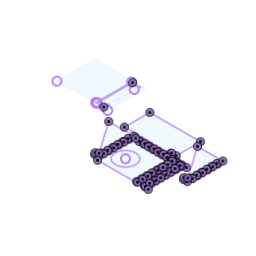
Verkefni2 (Autodesk Fusion 360 design; units mm, degrees)
Autodesk Fusion 360 part; units mm, degrees
note: some values were not read from the file. Chosen so that the rebuilt part matches the saved one: that a step has no effect.
sketch "haldari sketch" plane through (0, 0, 0) normal (1, 0, 0) x (0, 1, 0) in component "Fótur"
  line L0 (0, 0) -> (140, 0)
  line L1 (140, 0) -> (140, 100)
  line L2 (140, 100) -> (12.8948, 11)
  line L3 (12.8948, 11) -> (6.3582, 20.3352)
  line L4 (6.3582, 20.3352) -> (0, 15)
  line L5 (0, 15) -> (0, 0)
  dimension "d8" = 140
  dimension "d9" = 100
  dimension "d10" = 55
  dimension "d13" = 50
  dimension "d141" = 11
  dimension "d142" = 15
  constraint coincident L0.start L5.end
  constraint horizontal L0
  constraint perpendicular L0 L1
  constraint perpendicular L2 L3
  constraint perpendicular L0 L5
  measures "d8" distance of L0.start L0.end
  measures "d9" distance of L0.end L1.end
  measures "d10" angle of L1 L2
  measures "d13" angle of L4 L5
  measures "d141" distance of L0 L2.end
  measures "d142" distance of L0.start L4.end
extrude "Extrude6" add sketch "haldari sketch" along normal blind 4 makes body 1 in component "Fótur"
sketch "fingerhaldari sketch" plane through (4, 0, 0) normal (1, 0, 0) x (0, 1, 0) in component "Fótur"
  line L0 (0, 15) -> (0, 0)
  line L1 (0, 0) -> (140, 0)
  line L2 (140, 0) -> (140, 100)
  line L3 (140, 100) -> (12.8948, 11)
  line L4 (12.8948, 11) -> (6.3582, 20.3352)
  line L5 (6.3582, 20.3352) -> (0, 15)
  line L6 (90, 0) -> (90, 4)
  line L7 (90, 4) -> (0, 4)
  line L8 (0, 4) -> (0, 0)
  line L9 (20, 0) -> (40, 0)
  line L10 (40, 0) -> (40, 4)
  line L11 (40, 4) -> (20, 4)
  line L12 (20, 4) -> (20, 0)
  dimension "d72" = 4
  dimension "d73" = 20
  dimension "d79" = 20
  constraint vertical L6
  constraint horizontal L7
  constraint vertical L8
  constraint coincident L0.end L1.start
  constraint horizontal L9
  constraint vertical L10
  constraint horizontal L11
  constraint vertical L12
  constraint coincident L7 L10.end
  constraint coincident L1 L9.start
  measures "d72" distance of L0.end L7.end
  measures "d73" distance of L8 L12
  measures "d79" distance of L10.end L11.end
extrude "Extrude8" cut sketch "fingerhaldari sketch" against normal blind 4 contours L1 L7 L9 L10 L11 L12 bodies 1 in component "Fótur"
pattern_linear "R-Pattern2" count 3 spacing 40 along (0, 1, 0) of "Extrude8" in component "Fótur"
sketch "Sketch1" plane through (-1, 0, 0.1216) normal (0, 0, -1) x (1, 0, 0) in component "Botn"
  line L0 (32, -20) -> (36, -20)
  line L1 (36, -20) -> (36, 0)
  line L2 (36, 0) -> (32, 0)
  line L3 (32, 0) -> (32, -20)
  line L4 (-149, 4) -> (51, 4)
  line L5 (51, 4) -> (51, -146)
  line L6 (51, -146) -> (-149, -146)
  line L7 (-149, -146) -> (-149, 4)
  line L8 (1, 0) -> (1, -140)
  line L9 (1, 0) -> (5, 0)
  dimension "d96" = 200
  dimension "d97" = 150
  dimension "d98" = 150
  dimension "d99" = 4
  constraint horizontal L4
  constraint vertical L5
  constraint horizontal L6
  constraint vertical L7
  measures "d96" distance of L4.start L4.end
  measures "d97" distance of L4.start L6.end
  measures "d98" distance of L7 L8
  measures "d99" distance of L4 L9
extrude "Extrude1" add sketch "Sketch1" against normal blind 4 separate body makes body 2 in component "Botn"
combine "Combine1" operation cut target body 2 tool bodies 1 body 1 seen with x (1, 0, 0) y (0, 1, 0) z (0, 0, 1) at (31, 0, 0.1216) keep tools in component "Botn"
combine "Combine2" operation cut target body 2 tool bodies 1 keep tools in component "Botn"
combine "Combine3" operation cut target body 2 tool bodies 1 keep tools in component "Botn"
sketch "Sketch2" plane through (0, 0, 4.1216) normal (0, 0, 1) x (-1, 0, 0)
  line L0 (-31, -120) -> (-31, -140)
  line L1 (-35, -140) -> (-35, -120)
  line L2 (-35, -120) -> (-31, -120)
  line L3 (-31, -100) -> (-35, -100)
  line L4 (-35, -100) -> (-35, -80)
  line L5 (-35, -80) -> (-31, -80)
  line L6 (-31, -80) -> (-31, -100)
  line L7 (-31, -60) -> (-35, -60)
  line L8 (-35, -60) -> (-35, -40)
  line L9 (-35, -40) -> (-31, -40)
  line L10 (-31, -40) -> (-31, -60)
  line L11 (150, -146) -> (150, 4)
  line L12 (150, 4) -> (-50, 4)
  line L13 (-50, 4) -> (-50, -146)
  line L14 (-50, -146) -> (150, -146)
  line L15 (-31, -20) -> (-35, -20)
  line L16 (-35, -20) -> (-35, 0)
  line L17 (-4, -140) -> (-4, 0)
  line L18 (-4, 0) -> (0, 0)
  line L19 (0, 0) -> (0, -140)
  line L20 (0, -140) -> (-4, -140)
  line L21 (-31, -140) -> (-35, -140)
  line L22 (-35, 0) -> (-31, 0)
  line L23 (-31, 0) -> (-31, -20)
sketch "Sketch3" plane through (0, 146, 0) normal (0, 1, 0) x (-1, 0, 0)
  line L0 (-50, 0.1216) -> (150, 0.1216)
  line L1 (150, 0.1216) -> (150, 4.1216)
  line L2 (150, 4.1216) -> (-50, 4.1216)
  line L3 (-50, 4.1216) -> (-50, 0.1216)
  line L4 (-31.8182, 0.1216) -> (-13.6364, 0.1216)
  line L5 (-13.6364, 0.1216) -> (-13.6364, 4.1216)
  line L6 (-13.6364, 4.1216) -> (-31.8182, 4.1216)
  line L7 (-31.8182, 4.1216) -> (-31.8182, 0.1216)
  dimension "d133" = 18.1818
  dimension "d134" = 18.1818
  constraint horizontal L4
  constraint vertical L5
  constraint horizontal L6
  constraint vertical L7
  constraint coincident L2 L5.end
  constraint coincident L0 L4.start
  measures "d133" distance of L3 L7
  measures "d134" distance of L4.start L4.end
extrude "Extrude4" cut sketch "Sketch3" against normal blind 4 contours L0 L2 L4 L5 L6 L7 bodies 2 in component "Botn"
pattern_linear "R-Pattern2'" count 5 spacing 36.3636 along (-1, 0, 0) of "Extrude4" in component "Botn"
sketch "Sketch4" plane through (0, 0, 0.1216) normal (0, 0, -1) x (1, 0, 0)
  circle A0 centre (-100, -56) radius 40
  line L0 (-150, -146) -> (-150, 4)
  line L1 (-150, 4) -> (50, 4)
  dimension "d143" = 80
  dimension "d144" = 50
  dimension "d145" = 60
  measures "d143" diameter of A0
  measures "d144" distance of A0.centre L0
  measures "d145" distance of A0.centre L1
extrude "Extrude5" cut sketch "Sketch4" against normal blind 4 bodies 2 in component "Botn"
sketch "Sketch1 (2)" plane through (0, 146, 0) normal (0, 1, 0) x (-1, 0, 0) in component "Hlið"
  line L0 (-31.8182, 0.1216) -> (-31.8182, 4.1216)
  line L1 (-31.8182, 4.1216) -> (-50, 4.1216)
  line L2 (-50, 4.1216) -> (-50, 0.1216)
  line L3 (-50, 0.1216) -> (-31.8182, 0.1216)
  line L4 (-50, 0.1216) -> (150, 0.1216)
  line L5 (150, 0.1216) -> (150, 100.1216)
  line L6 (150, 100.1216) -> (-50, 100.1216)
  line L7 (-50, 100.1216) -> (-50, 0.1216)
  dimension "d148" = 200
  dimension "d149" = 100
  constraint horizontal L4
  constraint vertical L5
  constraint horizontal L6
  constraint vertical L7
  constraint coincident L2.end L3.start
  measures "d148" distance of L2.end L4.end
  measures "d149" distance of L2.end L6.end
extrude "Extrude1'" add sketch "Sketch1 (2)" against normal blind 4 separate body contours L0 L1 L4 L5 L6 L7 makes body 3 in component "Hlið"
combine "Combine1'" [no effect] in component "Hlið"
move_body "Move1" bodies 2 to x (1, 0, 0) y (0, 1, 0) z (0, 0, 1) at (70, -190, 0) in component "Botn"
move_body "Align1" bodies 1 to x (0, 0, 1) y (0, 1, 0) z (-1, 0, 0) at (50, 0, 4.1216) in component "Fótur"
move_body "Align2" bodies 1 to x (1, 0, 0) y (0, 1, 0) z (0, 0, 1) at (0, 0, -4.1216) in component "Fótur"
move_body "Align1'" bodies 3 to x (1, 0, 0) y (0, 0, -1) z (0, 1, 0) at (0, 91.8784, 146.1216) in component "Hlið"
move_body "Move1'" bodies 3 to x (1, 0, 0) y (0, 1, 0) z (0, 0, 1) at (0, -120, 0) in component "Hlið"
move_body "Move2" bodies 3 to x (1, 0, 0) y (0, 1, 0) z (0, 0, 1) at (10, 0, 0) in component "Hlið"
sketch "Sketch1 (3)" plane through (0, 0, 4.1216) normal (0, 0, 1) x (-1, 0, 0) in component "Cam Layer"
  circle A0 centre (-250, 134) radius 40
  line L0 (-381, 170) -> (-385, 170)
  line L1 (-385, 170) -> (-385, 190)
  line L2 (-385, 190) -> (-381, 190)
  line L3 (-381, 190) -> (-381, 170)
  line L4 (-236.3636, 44) -> (-236.3636, 48)
  line L5 (-236.3636, 48) -> (-218.1818, 48)
  line L6 (-218.1818, 48) -> (-218.1818, 44)
  line L7 (-218.1818, 44) -> (-200, 44)
  line L8 (-200, 44) -> (-200, 194)
  line L9 (-200, 194) -> (-400, 194)
  line L10 (-400, 194) -> (-400, 44)
  line L11 (-400, 44) -> (-381.8182, 44)
  line L12 (-381.8182, 44) -> (-381.8182, 48)
  line L13 (-381.8182, 48) -> (-363.6364, 48)
  line L14 (-363.6364, 48) -> (-363.6364, 44)
  line L15 (-363.6364, 44) -> (-345.4545, 44)
  line L16 (-345.4545, 44) -> (-345.4545, 48)
  line L17 (-345.4545, 48) -> (-327.2727, 48)
  line L18 (-327.2727, 48) -> (-327.2727, 44)
  line L19 (-327.2727, 44) -> (-309.0909, 44)
  line L20 (-309.0909, 44) -> (-309.0909, 48)
  line L21 (-309.0909, 48) -> (-290.9091, 48)
  line L22 (-290.9091, 48) -> (-290.9091, 44)
  line L23 (-290.9091, 44) -> (-272.7273, 44)
  line L24 (-272.7273, 44) -> (-272.7273, 48)
  line L25 (-272.7273, 48) -> (-254.5455, 48)
  line L26 (-254.5455, 48) -> (-254.5455, 44)
  line L27 (-254.5455, 44) -> (-236.3636, 44)
  line L28 (-381, 130) -> (-385, 130)
  line L29 (-385, 130) -> (-385, 150)
  line L30 (-385, 150) -> (-381, 150)
  line L31 (-381, 150) -> (-381, 130)
  line L32 (-381, 90) -> (-385, 90)
  line L33 (-385, 90) -> (-385, 110)
  line L34 (-385, 110) -> (-381, 110)
  line L35 (-381, 110) -> (-381, 90)
  line L36 (-381, 70) -> (-381, 50)
  line L37 (-381, 50) -> (-385, 50)
  line L38 (-385, 50) -> (-385, 70)
  line L39 (-385, 70) -> (-381, 70)
  line L40 (-354, 50) -> (-354, 190)
  line L41 (-354, 190) -> (-350, 190)
  line L42 (-350, 190) -> (-350, 50)
  line L43 (-350, 50) -> (-354, 50)
  line L44 (-190, 60) -> (-186, 60)
  line L45 (-186, 60) -> (-186, 80)
  line L46 (-186, 80) -> (-190, 80)
  line L47 (-190, 100) -> (-190, 80)
  line L48 (-190, 60) -> (-190, 40)
  line L49 (-190, 100) -> (-186, 100)
  line L50 (-186, 100) -> (-186, 120)
  line L51 (-186, 120) -> (-190, 120)
  line L52 (-190, 140) -> (-190, 120)
  line L53 (-190, 140) -> (-186, 140)
  line L54 (-186, 140) -> (-186, 160)
  line L55 (-186, 160) -> (-190, 160)
  line L56 (-190, 180) -> (-190, 160)
  line L57 (-175, 180) -> (-190, 180)
  line L58 (-169.6648, 173.6418) -> (-175, 180)
  line L59 (-179, 167.1052) -> (-169.6648, 173.6418)
  line L60 (-90, 40) -> (-179, 167.1052)
  line L61 (-190, 40) -> (-90, 40)
  line L62 (-140, 28) -> (-140, -72)
  line L63 (-140, -72) -> (-340, -72)
  line L64 (-340, -72) -> (-340, 24)
  line L65 (-321.8182, 24) -> (-340, 24)
  line L66 (-321.8182, 28) -> (-321.8182, 24)
  line L67 (-450, -30) -> (-446, -30)
  line L68 (-446, -30) -> (-446, -10)
  line L69 (-446, -10) -> (-450, -10)
  line L70 (-450, 10) -> (-450, -10)
  line L71 (-450, -30) -> (-450, -50)
  line L72 (-450, 10) -> (-446, 10)
  line L73 (-446, 10) -> (-446, 30)
  line L74 (-446, 30) -> (-450, 30)
  line L75 (-450, 50) -> (-450, 30)
  line L76 (-450, 50) -> (-446, 50)
  line L77 (-446, 50) -> (-446, 70)
  line L78 (-446, 70) -> (-450, 70)
  line L79 (-450, 90) -> (-450, 70)
  line L80 (-435, 90) -> (-450, 90)
  line L81 (-429.6648, 83.6418) -> (-435, 90)
  line L82 (-439, 77.1052) -> (-429.6648, 83.6418)
  line L83 (-350, -50) -> (-439, 77.1052)
  line L84 (-450, -50) -> (-350, -50)
  circle A1 centre (-250, 134) radius 40
  line L85 (-218.1818, 44) -> (-218.1818, 48)
  line L86 (-236.3636, 48) -> (-236.3636, 44)
  line L87 (-218.1818, 48) -> (-236.3636, 48)
  line L88 (-218.1818, 44) -> (-200, 44)
  line L89 (-254.5455, 44) -> (-236.3636, 44)
  line L90 (-254.5455, 44) -> (-254.5455, 48)
  line L91 (-272.7273, 48) -> (-272.7273, 44)
  line L92 (-254.5455, 48) -> (-272.7273, 48)
  line L93 (-290.9091, 44) -> (-290.9091, 48)
  line L94 (-309.0909, 48) -> (-309.0909, 44)
  line L95 (-290.9091, 48) -> (-309.0909, 48)
  line L96 (-290.9091, 44) -> (-272.7273, 44)
  line L97 (-327.2727, 44) -> (-309.0909, 44)
  line L98 (-327.2727, 44) -> (-327.2727, 48)
  line L99 (-345.4545, 48) -> (-345.4545, 44)
  line L100 (-327.2727, 48) -> (-345.4545, 48)
  line L101 (-363.6364, 44) -> (-363.6364, 48)
  line L102 (-381.8182, 48) -> (-381.8182, 44)
  line L103 (-363.6364, 48) -> (-381.8182, 48)
  line L104 (-363.6364, 44) -> (-345.4545, 44)
  line L105 (-400, 44) -> (-381.8182, 44)
  line L106 (-350, 110) -> (-354, 110)
  line L107 (-354, 130) -> (-350, 130)
  line L108 (-354, 50) -> (-350, 50)
  line L109 (-350, 50) -> (-350, 70)
  line L110 (-350, 170) -> (-350, 190)
  line L111 (-350, 130) -> (-350, 150)
  line L112 (-350, 90) -> (-350, 110)
  line L113 (-350, 70) -> (-354, 70)
  line L114 (-354, 90) -> (-350, 90)
  line L115 (-354, 70) -> (-354, 50)
  line L116 (-354, 110) -> (-354, 90)
  line L117 (-354, 150) -> (-354, 130)
  line L118 (-354, 190) -> (-354, 170)
  line L119 (-350, 150) -> (-354, 150)
  line L120 (-354, 170) -> (-350, 170)
  line L121 (-350, 190) -> (-354, 190)
  line L122 (-385, 50) -> (-381, 50)
  line L123 (-381, 130) -> (-381, 150)
  line L124 (-381, 90) -> (-381, 110)
  line L125 (-385, 110) -> (-385, 90)
  line L126 (-385, 150) -> (-385, 130)
  line L127 (-385, 70) -> (-385, 50)
  line L128 (-381, 70) -> (-385, 70)
  line L129 (-385, 90) -> (-381, 90)
  line L130 (-381, 50) -> (-381, 70)
  line L131 (-381, 110) -> (-385, 110)
  line L132 (-385, 130) -> (-381, 130)
  line L133 (-381, 150) -> (-385, 150)
  line L134 (-381, 190) -> (-385, 190)
  line L135 (-385, 190) -> (-385, 170)
  line L136 (-385, 170) -> (-381, 170)
  line L137 (-381, 170) -> (-381, 190)
  line L138 (-400, 194) -> (-400, 44)
  line L139 (-200, 194) -> (-400, 194)
  line L140 (-200, 44) -> (-200, 194)
  line L141 (-321.8182, 28) -> (-140, 28)
component "3D Model" placed x (1, 0, 0) y (0, 1, 0) z (0, 0, 1) at (0, 0, 0)
component "Cam Layer" placed x (1, 0, 0) y (0, 1, 0) z (0, 0, 1) at (0, 0, 0)
component "Fótur" placed x (1, 0, 0) y (0, 1, 0) z (0, 0, 1) at (0, 0, 0) in component "3D Model"
component "Fótur" placed x (1, 0, 0) y (0, 1, 0) z (0, 0, 1) at (31, 0, 0.1216) in component "3D Model"
component "Botn" placed x (1, 0, 0) y (0, 1, 0) z (0, 0, 1) at (0, 0, 0) in component "3D Model"
component "Hlið" placed x (1, 0, 0) y (0, 1, 0) z (0, 0, 1) at (0, 0, 0) in component "3D Model"
component "Fótur" placed x (1, 0, 0) y (0, 1, 0) z (0, 0, 1) at (140, -180, 0) in component "Cam Layer"
component "Fótur" placed x (1, 0, 0) y (0, 1, 0) z (0, 0, 1) at (400, -90, 0.1216) in component "Cam Layer"
component "Botn" placed x (1, 0, 0) y (0, 1, 0) z (0, 0, 1) at (280, 0, 0) in component "Cam Layer"
component "Hlið" placed x (1, 0, 0) y (0, 1, 0) z (0, 0, 1) at (280, 0, 0) in component "Cam Layer"
equation "haldaralengd = 140 mm"
equation "haldarahæð = 100 mm"
equation "endahæð = 30 mm"
equation "haldaraþykkt = 4 mm"
equation "fjarlægðmillihaldara = 35 mm"
equation "d8 = haldaralengd"
equation "d9 = haldarahæð"
equation "d10 = haldarafrahliðgraða"
equation "haldarafrahliðgraða = 55 deg"
equation "haldarafraendagraða = 50 deg"
equation "d13 = haldarafraendagraða"
equation "botnþykkt = 4 mm"
equation "botnlengd = 200 mm"
equation "botnhæð = 150 mm"
equation "hliðhæð = 100 mm"
equation "hliðlengd = 200 mm"
equation "hliðþykkt = 4 mm"
equation "armurfraendabotns = 150 mm"
equation "armurfrahliðbotns = 4 mm"
equation "hællarmurlengd = 20 mm"
equation "hællarmurhæð = 5 mm"
equation "hællfjarlægðfrahlið = 20 mm"
equation "d70 = haldaraþykkt"
equation "d72 = botnþykkt"
equation "d73 = lfingerw"
equation "lfingers = 3"
equation "wfingers = 5"
equation "hfingers = 3"
equation "lfingerw = haldaralengd / ( ( lfingers * 2 ) + 1 )"
equation "wfinger = hliðlengd / ( ( wfingers * 2 ) + 1 )"
equation "d79 = lfingerw"
equation "d86 = -haldaraþykkt"
equation "d88 = lfingers"
equation "d90 = -( haldaralengd - ( lfingerw * 3 ) )"
equation "d96 = botnlengd"
equation "d97 = botnhæð"
equation "d98 = armurfraendabotns"
equation "d99 = armurfrahliðbotns"
equation "d100 = -botnþykkt"
equation "hliðfraenda = 4 mm"
equation "þvermalcupholder = 80 mm"
equation "lengdcupholderfrahlið = 50 mm"
equation "lengdcupholderfraframhlið = 60 mm"
equation "d133 = wfinger"
equation "d134 = wfinger"
equation "d135 = -botnþykkt"
equation "d137 = wfingers"
equation "d139 = -( botnlengd - ( wfinger * 3 ) )"
equation "d143 = þvermalcupholder"
equation "d144 = lengdcupholderfrahlið"
equation "d145 = lengdcupholderfraframhlið"
equation "d146 = -botnþykkt"
equation "d148 = hliðlengd"
equation "d149 = hliðhæð"
equation "d150 = -hliðþykkt"
